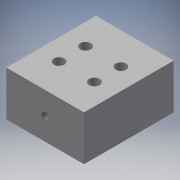
# Autodesk Inventor part: Mass 3
Saved by Autodesk Inventor 2016 (Build 200138000, 138)
## iProperties
Created: 2015-05-27
Part Number: Mass 3
Material: Steel, Mild
Document SubType Name: Modeling
Designer: Matthew Cheung
Density: 7.85 g/cm^3
Appearance: Steel
Mass: 416.076 g
Surface Area: 113.841 cm^2
Volume: 53.0034 cm^3
Author: Matthew Cheung
Autodesk Inventor part; units mm, degrees
ref_plane "YZ Plane" through (0, 0, 0) normal (1, 0, 0) x (0, 1, 0)
ref_plane "XZ Plane" through (0, 0, 0) normal (0, 1, 0) x (-1, 0, 0)
ref_plane "XY Plane" through (0, 0, 0) normal (0, 0, 1) x (1, 0, 0)
sketch "Sketch2" plane through (0, 0, 0) normal (0, 1, 0) x (-1, 0, 0)
  line L0 (-22, 25.4) -> (22, 25.4)
  line L1 (22, 25.4) -> (22, -25.4)
  line L2 (22, -25.4) -> (-22, -25.4)
  line L3 (-22, -25.4) -> (-22, 25.4)
  line L4 (-22, 25.4) -> (22, -25.4) construction
  line L5 (22, 25.4) -> (-22, -25.4) construction
  point P0 (0, 0)
  dimension "d0" = 50.8
  dimension "d1" = 44
  constraints: 12 end point, 2 midpoint, 2 parallel, 1 horizontal, 1 perpendicular
  measures "d0" distance of L0.end L1.end
  measures "d1" distance of L0.start L0.end
extrude "Extrusion1" add sketch "Sketch2" along normal blind 25.4
sketch "Sketch3" plane through (-22, 0, 25.4) normal (0, 0, 1) x (1, 0, 0)
  line L0 (0, 25.4) -> (44, 25.4) construction
  line L1 (0, 0) -> (44, 0) construction
  line L2 (44, 0) -> (44, 25.4) construction
  line L3 (44, 25.4) -> (0, 25.4) construction
  line L4 (0, 25.4) -> (0, 0) construction
  line L5 (0, 0) -> (44, 25.4) construction
  line L6 (44, 0) -> (0, 25.4) construction
  point P0 (22, 0)
  point P1 (22, 12.7)
  constraints: 12 end point, 2 midpoint, 2 parallel, 2 point on line, 1 horizontal, 1 perpendicular
hole "Hole1" at (0, 12.7, 25.4) direction (0, 0, -1) diameter 4.134 depth 19.05 tip angle 118 thread size "M5x0.8" class "6H" standard "ANSI Metric M Profile"
sketch "Sketch4" plane through (0, 25.4, 0) normal (0, 1, 0) x (1, 0, 0)
  line L0 (10, -7.5) -> (10, 7.5) construction
  line L1 (10, 7.5) -> (-10, 7.5) construction
  line L2 (-10, 7.5) -> (-10, -7.5) construction
  line L3 (-10, -7.5) -> (10, -7.5) construction
  line L4 (10, -7.5) -> (-10, 7.5) construction
  line L5 (10, 7.5) -> (-10, -7.5) construction
  circle A0 centre (-10, 7.5) radius 3
  circle A1 centre (10, 7.5) radius 3
  circle A2 centre (10, -7.5) radius 3
  circle A3 centre (-10, -7.5) radius 3
  point P0 (0, 0)
  dimension "d15" = 20
  dimension "d16" = 15
  dimension "d14" = 6
  dimension "d13" = 6
  dimension "d12" = 6
  dimension "d11" = 6
  constraints: 12 end point, 4 centre point, 4 coincident, 2 midpoint, 2 parallel, 1 perpendicular, 1 vertical
  measures "d15" distance of L0.end L1.end
  measures "d16" distance of L0.start L0.end
  measures "d14" diameter of A0
  measures "d13" diameter of A1
  measures "d12" diameter of A2
  measures "d11" diameter of A3
extrude "Extrusion2" cut sketch "Sketch4" against normal blind 5
sketch "Sketch5" plane through (-10, 20.4, 7.5) normal (0, 1, 0) x (1, 0, 0)
  circle A0 centre (0, 15) radius 3 projected
  circle A1 centre (20, 0) radius 3 projected
  circle A2 centre (20, 15) radius 3 projected
  point P0 (16, 18)
  point P1 (0, 0)
  constraints: 3 coincident
hole "Hole2" at (-10, 20.4, -7.5) at (-10, 20.4, 7.5) at (10, 20.4, 7.5) at (10, 20.4, -7.5) direction (0, -1, 0) diameter 3.5 end through all
body "Solid1"
